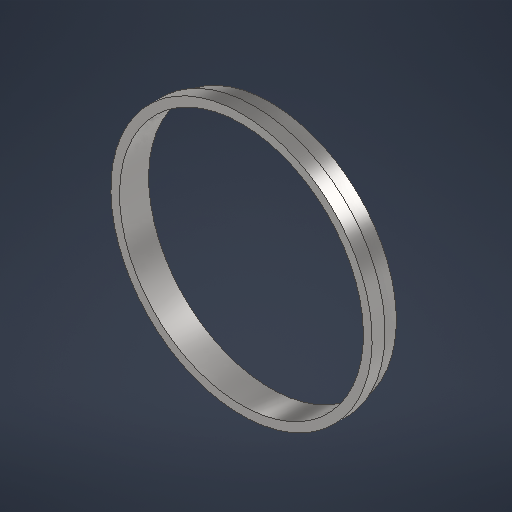
# Autodesk Inventor part: DiscoCorpoTurbina1
Saved by Autodesk Inventor 2026.2 (Build 302298010, 298A)
## iProperties
Created: 2026-04-30
Part Number: DiscoCorpoTurbina1
Material: Steel, Alloy
Document SubType Name: Modeling
Designer: Yan
Density: 7.73 g/cm^3
Appearance: Semi-Polished
Author: Yan
Autodesk Inventor part; units mm, degrees
ref_plane "YZ Plane" through (0, 0, 0) normal (1, 0, 0) x (0, 1, 0)
ref_plane "XZ Plane" through (0, 0, 0) normal (0, 1, 0) x (-1, 0, 0)
ref_plane "XY Plane" through (0, 0, 0) normal (0, 0, 1) x (1, 0, 0)
sketch "Sketch1" plane through (0, 0, 0) normal (1, 0, 0) x (0, 1, 0)
  line L0 (0, 0) -> (0, -90)
  line L1 (0, 0) -> (378, 0)
  line L2 (0, -90) -> (378, -90)
  line L3 (378, -90) -> (378, 0)
  line L4 (378, -90) -> (390, -90)
  line L5 (390, -90) -> (390, -40)
  line L6 (390, -40) -> (405, -40)
  line L7 (405, -40) -> (405, 0)
  line L8 (405, 0) -> (378, 0)
  dimension "d0" = 756
  dimension "d2" = 90
  dimension "d4" = 780
  dimension "d5" = 40
  dimension "d6" = 810
  constraints: 18 end point, 4 perpendicular, 3 horizontal, 2 vertical
  measures "d0" diameter of L3 L0
  measures "d2" distance between parallel lines of L2 L1
  measures "d4" diameter of L5 L0
  measures "d5" distance of L6.end L7.end
  measures "d6" diameter of L7 L0
revolve "Revolution1" add sketch "Sketch1" angle 360 about axis through (0, 0, 0) along (0, 0, -1) contours L8 L7 L6 L5 L4 L3
body "Solid1"
